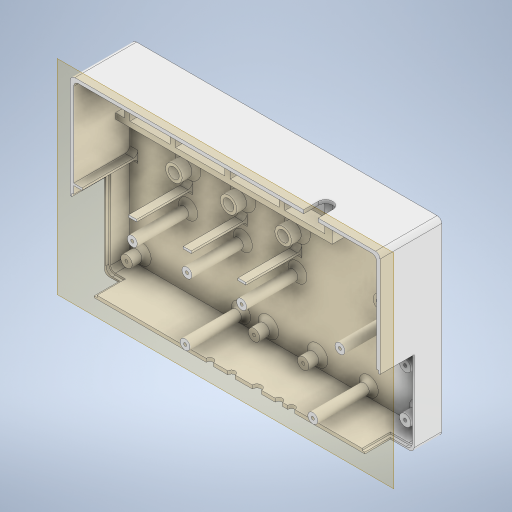
# Autodesk Inventor part: RV_ES_Bottom
Saved by Autodesk Inventor 2023.3 (Build 273359000, 359)
## iProperties
Created: 2023-07-31
Part Number: RV_ES_Bottom
Material: PC/ABS Plastic
Document SubType Name: Modeling
Designer: atrus
Density: 0.357273 g/cm^3
Appearance: Smooth - White
Author: atrus
Autodesk Inventor part; units mm, degrees
ref_plane "YZ Plane" through (0, 0, 0) normal (1, 0, 0) x (0, 1, 0)
ref_plane "XZ Plane" through (0, 0, 0) normal (0, 1, 0) x (-1, 0, 0)
ref_plane "XY Plane" through (0, 0, 0) normal (0, 0, 1) x (1, 0, 0)
sketch "Sketch1" plane through (0, 0, 0) normal (0, 0, 1) x (1, 0, 0)
  line L0 (0, 0) -> (215.9, 0)
  line L1 (215.9, 0) -> (215.9, 132.08)
  line L2 (215.9, 132.08) -> (0, 132.08)
  line L3 (0, 132.08) -> (0, 0)
  dimension "d0" = 215.9
  dimension "d1" = 132.08
  constraints: 8 end point, 2 parallel, 1 horizontal, 1 perpendicular
  measures "d0" distance of L1.end L2.end
  measures "d1" distance of L0.end L1.end
extrude "BasePlate" add sketch "Sketch1" along normal blind 4
sketch "Sketch2" plane through (0, 0, 4) normal (0, 0, 1) x (1, 0, 0)
  circle A0 centre (10.16, 10.16) radius 1.7 construction
  circle A1 centre (99.06, 10.16) radius 1.7 construction
  circle A2 centre (133.35, 10.16) radius 1.7 construction
  circle A3 centre (204.47, 11.43) radius 1.7 construction
  circle A4 centre (156.21, 123.19) radius 1.7 construction
  circle A5 centre (123.19, 123.19) radius 1.7 construction
  circle A6 centre (80.01, 123.19) radius 1.7 construction
  circle A7 centre (46.99, 123.134) radius 1.7 construction
  circle A8 centre (10.16, 10.16) radius 4
  circle A9 centre (99.06, 10.16) radius 4
  circle A10 centre (133.35, 10.16) radius 4
  circle A11 centre (204.47, 11.43) radius 4
  circle A12 centre (156.21, 123.19) radius 4
  circle A13 centre (123.19, 123.19) radius 4
  circle A14 centre (80.01, 123.19) radius 4
  circle A15 centre (46.99, 123.134) radius 4
  circle A16 centre (8.89, 123.19) radius 1.7 construction
  circle A17 centre (8.89, 123.19) radius 4
  circle A18 centre (204.47, 44.45) radius 4
  circle A19 centre (204.47, 44.45) radius 1.7 construction
  point P0 (0, 0)
  dimension "d4" = 8
  constraints: 11 centre point, 9 equal radius, 1 coincident, 2 other
  measures "d4" diameter of A8
ref_plane "Work Plane1" through (212.09, 125.73, 14) normal (0, 0, -1) x (0.0000001, -1, 0)
extrude "PCB Screw Bosses" add sketch "Sketch2" along normal up to surface (10 mm away)
sketch "Sketch3" plane through (0, 0, 4) normal (0, 0, 1) x (1, 0, 0)
  line L0 (0, 0) -> (215.9, 0)
  line L1 (215.9, 0) -> (215.9, 132.08)
  line L2 (215.9, 132.08) -> (0, 132.08)
  line L3 (0, 132.08) -> (0, 0)
  line L4 (213.487, 129.667) -> (213.487, 2.413)
  line L5 (213.487, 2.413) -> (2.413, 2.413)
  line L6 (2.413, 2.413) -> (2.413, 129.667)
  line L7 (2.413, 129.667) -> (213.487, 129.667)
  point P0 (0, 132.08)
  point P1 (215.9, 0)
  dimension "d7" = 2.413
  constraints: 16 end point, 4 parallel, 2 perpendicular, 1 horizontal, 3 other
  measures "d7" distance between parallel lines of L1 L4
extrude "OuterCaseWall" add sketch "Sketch3" along normal blind 15.24
sketch "Sketch4" plane through (0, 0, 4) normal (0, 0, 1) x (1, 0, 0)
  line L0 (2.413, 129.667) -> (2.413, 2.413) projected
  line L1 (153.543, 93.8851) -> (153.543, 92.202)
  line L2 (153.543, 92.202) -> (2.413, 92.202)
  line L3 (2.413, 92.202) -> (2.413, 96.012)
  line L4 (153.543, 115.9189) -> (153.543, 117.602)
  line L5 (153.543, 117.602) -> (2.413, 117.602)
  line L6 (2.413, 117.602) -> (2.413, 113.792)
  line L7 (2.413, 129.667) -> (213.487, 129.667) projected
  line L8 (44.323, 96.012) -> (44.323, 113.792)
  line L9 (40.513, 113.792) -> (40.513, 96.012)
  line L10 (82.423, 96.012) -> (82.423, 113.792)
  line L11 (78.613, 113.792) -> (78.613, 96.012)
  line L12 (120.523, 96.012) -> (120.523, 113.792)
  line L13 (116.713, 113.792) -> (116.713, 96.012)
  line L14 (148.463, 113.792) -> (148.463, 96.012)
  line L15 (153.543, 93.5809) -> (153.543, 115.9189)
  line L16 (8.763, 96.012) -> (8.763, 113.792)
  line L17 (12.573, 113.792) -> (12.573, 96.012)
  line L18 (2.413, 96.012) -> (8.763, 96.012)
  line L19 (12.573, 96.012) -> (40.513, 96.012)
  line L20 (44.323, 96.012) -> (78.613, 96.012)
  line L21 (44.323, 113.792) -> (78.613, 113.792)
  line L22 (2.413, 113.792) -> (8.763, 113.792)
  line L23 (12.573, 113.792) -> (40.513, 113.792)
  line L24 (82.423, 113.792) -> (116.713, 113.792)
  line L25 (120.523, 113.792) -> (148.463, 113.792)
  line L26 (82.423, 96.012) -> (116.713, 96.012)
  line L27 (120.523, 96.012) -> (148.463, 96.012)
  point P0 (0, 0)
  point P1 (2.413, 115.697)
  point P2 (2.413, 94.107)
  point P3 (2.413, 117.602)
  point P4 (2.413, 92.202)
  point P5 (153.543, 93.8851)
  dimension "d10" = 13.97
  dimension "d11" = 21.59
  dimension "d12" = 3.81
  dimension "d13" = 6.35
  dimension "d14" = 151.13
  dimension "d15" = 3.81
  dimension "d16" = 3.81
  dimension "d17" = 3.81
  dimension "d18" = 3.81
  dimension "d19" = 3.81
  dimension "d20" = 27.94
  dimension "d21" = 34.29
  dimension "d22" = 34.29
  dimension "d23" = 27.94
  constraints: 52 end point, 17 parallel, 10 horizontal, 10 perpendicular, 8 collinear, 4 equal length, 2 midpoint, 2 point on line
  measures "d10" distance from line of point (2.413, 115.697) L7
  measures "d11" distance of point (2.413, 115.697) point (2.413, 94.107)
  measures "d12" distance between parallel lines of L17 L16
  measures "d13" distance between parallel lines of L0 L16
  measures "d14" distance of L4.end L5.end
  measures "d15" distance between parallel lines of L9 L8
  measures "d16" distance between parallel lines of L10 L11
  measures "d17" distance between parallel lines of L12 L13
  measures "d18" distance between parallel lines of L5 L23
  measures "d19" distance between parallel lines of L2 L19
  measures "d20" distance between parallel lines of L17 L9
  measures "d21" distance between parallel lines of L8 L11
  measures "d22" distance between parallel lines of L10 L13
  measures "d23" distance between parallel lines of L14 L12
extrude "ReceptBottomRibs" add sketch "Sketch4" along normal up to surface (10 mm away) contours L5 L4 L15 L1 L2 L0 L18 L16 L22
sketch "Sketch5" plane through (0, 0, 4) normal (0, 0, 1) x (1, 0, 0)
  line L0 (54.2784, 65.754) -> (31.8784, 65.754) construction
  line L1 (31.8784, 68.754) -> (54.2784, 68.754) construction
  line L2 (77.7501, 59.2541) -> (77.7501, 75.2541) construction
  line L3 (85.3501, 75.2541) -> (85.3501, 59.2541) construction
  line L4 (70.08, 68.754) -> (92.48, 68.754) construction
  line L5 (92.48, 65.754) -> (70.08, 65.754) construction
  line L6 (3.81, 68.5117) -> (19.05, 68.5117) construction
  line L7 (19.0355, 65.9695) -> (3.81, 65.9695) construction
  line L8 (9.1501, 75.2541) -> (9.1501, 59.2541) construction
  line L9 (39.6501, 59.2541) -> (39.6501, 75.2541) construction
  line L10 (47.2501, 75.2541) -> (47.2501, 59.2541) construction
  line L11 (115.8501, 59.2541) -> (115.8501, 75.2541) construction
  line L12 (123.4501, 75.2541) -> (123.4501, 59.2541) construction
  line L13 (130.58, 65.754) -> (108.18, 65.754) construction
  line L14 (108.18, 68.754) -> (130.58, 68.754) construction
  line L15 (172.95, 68.754) -> (195.35, 68.754) construction
  line L16 (195.35, 65.754) -> (172.95, 65.754) construction
  line L17 (182.51, 53.454) -> (182.51, 105.854) construction
  line L18 (2.413, 92.202) -> (2.413, 2.413) projected
  line L19 (2.413, 68.0117) -> (8.1501, 68.0117)
  line L20 (8.1501, 68.0117) -> (8.1501, 66.4695)
  line L21 (8.1501, 66.4695) -> (2.413, 66.4695)
  line L22 (2.413, 66.4695) -> (2.413, 68.0117)
  line L23 (40.6501, 68.0117) -> (46.2501, 68.0117)
  line L24 (46.2501, 68.0117) -> (46.2501, 66.4695)
  line L25 (46.2501, 66.4695) -> (40.6501, 66.4695)
  line L26 (40.6501, 66.4695) -> (40.6501, 68.0117)
  line L27 (78.7501, 68.0117) -> (84.3501, 68.0117)
  line L28 (84.3501, 68.0117) -> (84.3501, 66.4695)
  line L29 (84.3501, 66.4695) -> (78.7501, 66.4695)
  line L30 (78.7501, 66.4695) -> (78.7501, 68.0117)
  line L31 (116.8501, 68.0117) -> (122.4501, 68.0117)
  line L32 (122.4501, 68.0117) -> (122.4501, 66.4695)
  line L33 (122.4501, 66.4695) -> (116.8501, 66.4695)
  line L34 (116.8501, 66.4695) -> (116.8501, 68.0117)
  line L35 (183.51, 66.4695) -> (194.85, 66.4695)
  line L36 (194.85, 66.4695) -> (194.85, 68.0117)
  line L37 (194.85, 68.0117) -> (183.51, 68.0117)
  line L38 (183.51, 68.0117) -> (183.51, 66.4695)
  point P0 (0, 0)
  dimension "d26" = 0.5
  dimension "d27" = 0.5
  dimension "d28" = 1
  dimension "d29" = 1
  dimension "d30" = 1
  dimension "d31" = 1
  dimension "d32" = 1
  dimension "d33" = 1
  dimension "d34" = 1
  dimension "d35" = 1
  dimension "d36" = 0.5
  constraints: 40 end point, 10 parallel, 9 point on line, 5 horizontal, 5 perpendicular
  measures "d26" distance between parallel lines of L6 L19
  measures "d27" distance between parallel lines of L7 L21
  measures "d28" distance between parallel lines of L8 L20
  measures "d29" distance between parallel lines of L9 L26
  measures "d30" distance from line of L10 L24.end
  measures "d31" distance between parallel lines of L2 L30
  measures "d32" distance between parallel lines of L3 L28
  measures "d33" distance between parallel lines of L11 L34
  measures "d34" distance between parallel lines of L12 L32
  measures "d35" distance between parallel lines of L17 L38
  measures "d36" distance from line of L15.end L36
ref_plane "Top Of Case" through (17.5673, 114.3074, 42.9916) normal (0, 0, 1) x (1, 0, 0)
ref_plane "Offset Top Of Case" through (17.5673, 114.3074, 42.7916) normal (0, 0, 1) x (1, 0, 0)
extrude "Barriers" add sketch "Sketch5" along normal up to surface (38.9916 mm away) contours L19 L20 L21 L18 | L23 L24 L25 L26 | L27 L28 L29 L30 | L31 L32 L33 L34
sketch "Sketch6" plane through (0, 0, 4) normal (0, 0, 1) x (1, 0, 0)
  circle A0 centre (29.21, 123.19) radius 3.75 projected
  circle A1 centre (90.17, 123.19) radius 3.75 projected
  circle A2 centre (113.03, 123.19) radius 3.75 projected
  circle A3 centre (181.61, 123.19) radius 3.75 projected
  circle A4 centre (187.96, 73.66) radius 3.75 projected
  circle A5 centre (119.38, 80.01) radius 3.75 projected
  circle A6 centre (81.28, 80.01) radius 3.75 projected
  circle A7 centre (43.18, 80.01) radius 3.75 projected
  circle A8 centre (29.21, 123.19) radius 5.75
  circle A9 centre (90.17, 123.19) radius 5.75
  circle A10 centre (113.03, 123.19) radius 5.75
  circle A11 centre (181.61, 123.19) radius 5.75
  circle A12 centre (187.96, 73.66) radius 5.75
  circle A13 centre (119.38, 80.01) radius 5.75
  circle A14 centre (81.28, 80.01) radius 5.75
  circle A15 centre (43.18, 80.01) radius 5.75
  dimension "d52" = 2
  constraints: 8 centre point, 7 equal radius
  measures "d52" radial gap between concentric circles of A0 A8
extrude "HVSideBosses" add sketch "Sketch6" along normal up to surface (10 mm away)
sketch "Sketch7" plane through (0, 0, 0) normal (0, 0, -1) x (-1, 0, 0)
  circle A0 centre (-81.28, 80.01) radius 3.75 projected
  circle A1 centre (-29.21, 123.19) radius 3.75 projected
  circle A2 centre (-90.17, 123.19) radius 3.75 projected
  circle A3 centre (-113.03, 123.19) radius 3.75 projected
  circle A4 centre (-181.61, 123.19) radius 3.75 projected
  circle A5 centre (-43.18, 80.01) radius 3.75 construction
  circle A6 centre (-81.28, 80.01) radius 3.75 construction
  circle A7 centre (-119.38, 80.01) radius 3.75 construction
  circle A8 centre (-187.96, 73.66) radius 3.75 construction
  point P0 (0, 0)
  constraints: 5 coincident
hole "HotSideHoles" at (81.28, 80.01, 0) at (29.21, 123.19, 0) at (90.17, 123.19, 0) at (113.03, 123.19, 0) at (181.61, 123.19, 0) at (43.18, 80.01, 0) at (119.38, 80.01, 0) at (187.96, 73.66, 0) direction (0, 0, 1) diameter 3.2766 end through all counterbore diameter 7.62 counterbore depth 3 clearance for "Flat Head Machine Screw (82)" size "#4" standard "Ansi Unified Screw Threads"
chamfer "HotSideHoleChamfer" distance 2.032 angle 45 8 edges at (81.28, 76.2, 3) (90.17, 119.38, 3) (113.03, 119.38, 3) (181.61, 119.38, 3) (29.21, 119.38, 3) (187.96, 69.85, 3) (119.38, 76.2, 3) (43.18, 76.2, 3)
sketch "Sketch8" plane through (0, 0, 4) normal (0, 0, 1) x (1, 0, 0)
  circle A0 centre (169.052, 9.398) radius 3.45
  circle A1 centre (80.01, 9.398) radius 3.45
  circle A2 centre (81.28, 53.34) radius 3.45
  circle A3 centre (119.38, 53.34) radius 3.45
  circle A4 centre (187.96, 60.96) radius 3.45
  circle A5 centre (43.18, 53.34) radius 3.45
  circle A6 centre (169.052, 9.398) radius 3.75 projected
  circle A7 centre (187.96, 60.96) radius 3.75 projected
  circle A8 centre (119.38, 53.34) radius 3.75 projected
  circle A9 centre (81.28, 53.34) radius 3.75 projected
  circle A10 centre (43.18, 53.34) radius 3.75 projected
  circle A11 centre (80.01, 9.398) radius 3.75 projected
  point P0 (0, 0)
  dimension "d53" = 0.3
  constraints: 6 centre point, 6 coincident, 5 equal radius
  measures "d53" radial gap between concentric circles of A10 A5
extrude "LogicSideBosses" add sketch "Sketch8" along normal up to surface (38.9916 mm away) contours A0 | A1 | A2 | A3 | A4 | A5
sketch "Sketch9" plane through (81.28, 53.34, 42.9916) normal (0, 0, 1) x (1, 0, 0)
  circle A0 centre (-38.1, 0) radius 3.45 construction
  circle A1 centre (0, 0) radius 3.45 construction
  circle A2 centre (38.1, 0) radius 3.45 construction
  circle A3 centre (106.68, 7.62) radius 3.45 construction
  circle A4 centre (87.772, -43.942) radius 3.45 construction
  circle A5 centre (17.78, -43.18) radius 4
  circle A6 centre (-1.27, -43.942) radius 3.45 construction
  point P0 (-81.28, -53.34)
  constraints: 1 centre point
hole "LogicSideHoles" at (43.18, 53.34, 42.9916) at (81.28, 53.34, 42.9916) at (119.38, 53.34, 42.9916) at (187.96, 60.96, 42.9916) at (169.052, 9.398, 42.9916) at (80.01, 9.398, 42.9916) direction (0, 0, -1) diameter 2.1565 depth 17.78 tip angle 118 thread size "4-40 UNC" class "2B" standard "ANSI Unified Screw Threads"
fillet "Fillet1" radius 3.175 29 edges at (39.73, 53.34, 4) (77.83, 53.34, 4) (115.93, 53.34, 4) (76.56, 9.398, 4) (165.602, 9.398, 4) (184.51, 60.96, 4) (119.6501, 66.4695, 4) (81.5501, 66.4695, 4) (43.4501, 66.4695, 4) (113.63, 80.01, 4) (119.6501, 68.0117, 4) (75.53, 80.01, 4) (81.5501, 68.0117, 4) (37.43, 80.01, 4) (43.4501, 68.0117, 4) (5.2815, 68.0117, 4) (5.2815, 66.4695, 4) (42.99, 123.134, 4) (76.01, 123.19, 4) (119.19, 123.19, 4) (4.89, 123.19, 4) (175.86, 123.19, 4) (152.21, 123.19, 4) (29.21, 128.94, 4) (6.16, 10.16, 4) (95.06, 10.16, 4) (129.35, 10.16, 4) (200.47, 11.43, 4) (200.47, 44.45, 4)
sketch "Sketch10" plane through (46.99, 123.134, 14) normal (0, 0, 1) x (1, 0, 0)
  circle A0 centre (-38.1, 0.056) radius 4 projected
  circle A1 centre (0, 0) radius 4 projected
  circle A2 centre (33.02, 0.056) radius 4 projected
  circle A3 centre (76.2, 0.056) radius 4 projected
  circle A4 centre (109.22, 0.056) radius 4 projected
  circle A5 centre (157.48, -111.704) radius 4 projected
  circle A6 centre (86.36, -112.974) radius 4 projected
  circle A7 centre (52.07, -112.974) radius 4 projected
  circle A8 centre (-36.83, -112.974) radius 4 projected
  line L0 (-44.577, -120.721) -> (166.497, -120.721) projected
  line L1 (166.497, -120.721) -> (166.497, 6.533) projected
  line L2 (166.497, 6.533) -> (140.7604, 6.533) projected
  line L3 (106.553, -6.6049) -> (106.553, -30.932) projected
  line L4 (106.553, -30.932) -> (-44.577, -30.932) projected
  line L5 (-44.577, -30.932) -> (-44.577, -51.9474) projected
  line L6 (-38.8399, -51.9474) -> (-38.8399, -59.8395) projected
  line L7 (-44.577, -59.8395) -> (-44.577, -120.721) projected
  line L8 (37.3601, -51.9474) -> (37.3601, -59.8395) projected
  line L9 (31.7601, -59.8395) -> (31.7601, -51.9474) projected
  circle A9 centre (140.97, -49.474) radius 5.75 projected
  line L10 (75.4601, -51.9474) -> (75.4601, -59.8395) projected
  line L11 (69.8601, -59.8395) -> (69.8601, -51.9474) projected
  line L12 (-0.7399, -51.9474) -> (-0.7399, -59.8395) projected
  line L13 (-6.3399, -59.8395) -> (-6.3399, -51.9474) projected
  circle A10 centre (157.48, -78.684) radius 1.7 projected
  line L14 (-44.577, 6.533) -> (-44.577, 3.1429) projected
  line L15 (-33.5995, -5.532) -> (-24.7392, -5.532) projected
  line L16 (-10.8208, -5.532) -> (-4.5692, -5.532) projected
  line L17 (4.5692, -5.532) -> (28.5195, -5.532) projected
  arc A11 (44.5353, -5.532) -> (39.0064, 4.0112) centre (43.18, 0.056) ccw projected
  line L18 (44.5353, -5.532) -> (64.6847, -5.532) projected
  arc A12 (70.2136, 4.0112) -> (64.6847, -5.532) centre (66.04, 0.056) ccw projected
  line L19 (-38.227, -9.342) -> (-44.577, -9.342) projected
  line L20 (-44.577, -27.122) -> (-38.227, -27.122) projected
  line L21 (-38.227, -27.122) -> (-38.227, -9.342) projected
  line L22 (-44.577, -3.0309) -> (-44.577, -5.532) projected
  line L23 (-44.577, -9.342) -> (-44.577, -27.122) projected
  arc A13 (29.9331, 6.533) -> (28.5195, -5.532) centre (33.02, 0.056) ccw projected
  line L24 (29.9331, 6.533) -> (2.9666, 6.533) projected
  arc A14 (4.5692, -5.532) -> (2.9666, 6.533) centre (0, 0) ccw projected
  arc A15 (73.1131, 6.533) -> (70.2136, 4.0112) centre (76.2, 0.056) ccw projected
  line L25 (73.1131, 6.533) -> (36.1069, 6.533) projected
  arc A16 (39.0064, 4.0112) -> (36.1069, 6.533) centre (33.02, 0.056) ccw projected
  arc A17 (-41.1869, 6.533) -> (-44.577, 3.1429) centre (-38.1, 0.056) ccw projected
  line L26 (-41.1869, 6.533) -> (-44.577, 6.533) projected
  arc A18 (-44.577, -3.0309) -> (-42.6005, -5.532) centre (-38.1, 0.056) ccw projected
  line L27 (-44.577, -5.532) -> (-42.6005, -5.532) projected
  arc A19 (-10.8208, -5.532) -> (-11.6396, 6.533) centre (-17.78, 0.056) ccw projected
  arc A20 (-2.9666, 6.533) -> (-4.5692, -5.532) centre (0, 0) ccw projected
  line L28 (-2.9666, 6.533) -> (-11.6396, 6.533) projected
  arc A21 (-23.9204, 6.533) -> (-24.7392, -5.532) centre (-17.78, 0.056) ccw projected
  line L29 (-23.9204, 6.533) -> (-35.0131, 6.533) projected
  arc A22 (-33.5995, -5.532) -> (-35.0131, 6.533) centre (-38.1, 0.056) ccw projected
  circle A23 centre (-36.83, -112.974) radius 7.175 projected
  arc A24 (128.4796, 6.533) -> (140.7604, 6.533) centre (134.62, 0.056) ccw projected
  line L30 (128.4796, 6.533) -> (112.3069, 6.533) projected
  arc A25 (106.553, -6.6049) -> (112.3069, 6.533) centre (109.22, 0.056) ccw projected
  line L31 (-38.8399, -51.9474) -> (-44.577, -51.9474) projected
  line L32 (-44.577, -59.8395) -> (-38.8399, -59.8395) projected
  line L33 (31.7601, -59.8395) -> (37.3601, -59.8395) projected
  line L34 (32.9468, -51.9474) -> (31.7601, -51.9474) projected
  arc A26 (35.6332, -51.9474) -> (32.9468, -51.9474) centre (34.29, -43.124) ccw projected
  line L35 (37.3601, -51.9474) -> (35.6332, -51.9474) projected
  circle A27 centre (140.97, -62.174) radius 6.625 projected
  line L36 (69.8601, -59.8395) -> (75.4601, -59.8395) projected
  line L37 (71.0467, -51.9474) -> (69.8601, -51.9474) projected
  arc A28 (73.7333, -51.9474) -> (71.0467, -51.9474) centre (72.39, -43.124) ccw projected
  line L38 (75.4601, -51.9474) -> (73.7333, -51.9474) projected
  line L39 (-6.3399, -59.8395) -> (-0.7399, -59.8395) projected
  line L40 (-5.1533, -51.9474) -> (-6.3399, -51.9474) projected
  arc A29 (-2.4667, -51.9474) -> (-5.1533, -51.9474) centre (-3.81, -43.124) ccw projected
  line L41 (-0.7399, -51.9474) -> (-2.4667, -51.9474) projected
  point P0 (-46.99, -123.134)
hole "PCBMountHoles" at (46.99, 123.134, 14) at (8.89, 123.19, 14) at (80.01, 123.19, 14) at (123.19, 123.19, 14) at (156.21, 123.19, 14) at (10.16, 10.16, 14) at (99.06, 10.16, 14) at (133.35, 10.16, 14) at (204.47, 11.43, 14) at (204.47, 44.45, 14) direction (0, 0, -1) diameter 2.1565 end through all thread size "4-40 UNC" class "2B" standard "ANSI Unified Screw Threads"
sketch "Sketch11" plane through (0, 0, 19.24) normal (0, 0, 1) x (1, 0, 0)
  line L0 (2.413, 59.2541) -> (2.413, 129.667) projected
  line L1 (2.413, 59.2541) -> (2.413, 129.667)
  line L2 (2.413, 129.667) -> (213.487, 129.667) projected
  line L3 (2.413, 129.667) -> (213.487, 129.667)
  line L4 (213.487, 129.667) -> (213.487, 59.2541)
  line L5 (213.487, 129.667) -> (213.487, 2.413) projected
  line L6 (215.9, 0) -> (215.9, 132.08) projected
  line L7 (215.9, 59.2541) -> (215.9, 132.08)
  line L8 (215.9, 132.08) -> (0, 132.08)
  line L9 (0, 132.08) -> (0, 59.2541)
  line L10 (0, 132.08) -> (0, 0) projected
  line L11 (2.413, 59.2541) -> (0, 59.2541)
  line L12 (213.487, 59.2541) -> (215.9, 59.2541)
  line L13 (9.1501, 59.2541) -> (39.6501, 59.2541) construction
  point P0 (2.413, 66.4695)
  point P1 (1.2065, 59.2541)
  constraints: 16 end point, 3 point on line, 2 collinear, 2 horizontal, 2 horizontal alignment, 2 vertical, 1 midpoint, 1 perpendicular
extrude "HV Upper Wall" add sketch "Sketch11" along normal up to surface (23.7516 mm away)
sketch "Sketch12" plane through (0, 132.08, 0) normal (0, 1, 0) x (1, 0, 0)
  line L0 (213.487, -42.9916) -> (2.413, -42.9916) projected
  line L1 (172.72, -42.9916) -> (172.72, -32.7516)
  line L2 (167.72, -27.7516) -> (167.72, -27.7516)
  line L3 (162.72, -32.7516) -> (162.72, -42.9916)
  line L4 (215.9, 0) -> (215.9, -42.9916) projected
  arc A0 (167.72, -27.7516) -> (162.72, -32.7516) centre (167.72, -32.7516) ccw
  arc A1 (172.72, -32.7516) -> (167.72, -27.7516) centre (167.72, -32.7516) ccw
  point P0 (0, 0)
  point P1 (172.72, -27.7516)
  point P2 (162.72, -27.7516)
  point P3 (172.72, -37.8716)
  dimension "d74" = 10
  dimension "d75" = 43.18
  dimension "d76" = 15.24
  dimension "d77" = 5
  constraints: 6 end point, 6 point on line, 4 point on circle, 4 tangent, 2 centre point, 2 perpendicular, 1 concentric, 1 midpoint, 1 vertical
  measures "d74" distance of point (172.72, -27.752) point (162.72, -27.752)
  measures "d75" distance from line of L4 point (172.72, -37.872)
  measures "d76" distance of point (162.72, -27.752) L3.end
  measures "d77" radius of A0
extrude "Cord cut" cut sketch "Sketch12" against normal blind 25.4
fillet "HV Corner Fillets" radius 3.175 4 edges at (0, 132.08, 21.4958) (213.487, 129.667, 23.4958) (215.9, 132.08, 21.4958) (2.413, 129.667, 23.4958)
sketch "Sketch13" plane through (187.96, 73.66, 14) normal (0, 0, 1) x (1, 0, 0)
  line L0 (-65.5099, -5.6483) -> (-65.5099, -7.1905) construction
  line L1 (25.527, -71.247) -> (25.527, 52.832) construction
  line L2 (-4.3589, -6.075) -> (-4.3589, -3.75)
  line L3 (-4.3589, -3.75) -> (4.3589, -3.75)
  line L4 (4.3589, -3.75) -> (4.3589, -6.075)
  line L5 (4.3589, -6.075) -> (-4.3589, -6.075)
  circle A0 centre (0, 0) radius 5.75 projected
  circle A1 centre (0, 0) radius 3.75 projected
  circle A2 centre (0, -12.7) radius 6.625 construction
  point P0 (-187.96, -73.66)
  point P1 (0, -3.75)
  constraints: 8 end point, 2 point on circle, 2 vertical, 1 midpoint, 1 parallel, 1 perpendicular, 1 tangent, 1 vertical alignment, 1 other
extrude "BossCutPowerSupply" cut sketch "Sketch13" against normal up to surface (10 mm away) contours L2 A0 L4 L5 | L3 A0 picked at (2.5581, -4.066)
fillet "LgicCornerFillets" radius 3.175 4 edges at (0, 0, 9.62) (215.9, 0, 9.62) (2.413, 2.413, 11.62) (213.487, 2.413, 11.62)
sketch "Sketch14" plane through (0, 0, 19.24) normal (0, 0, 1) x (1, 0, 0)
  circle A0 centre (80.01, 9.398) radius 1.0782 construction
  circle A1 centre (80.01, 9.398) radius 3.45 construction
  line L0 (151.92, 16.9397) -> (151.92, 21.3401) construction
  line L1 (84.975, 21.3101) -> (84.975, 16.9097) construction
  line L2 (5.588, 2.413) -> (210.312, 2.413) projected
  line L3 (3.175, 0) -> (212.725, 0) projected
  line L4 (10.668, 2.413) -> (199.39, 2.413)
  line L5 (199.39, 2.413) -> (199.39, 0)
  line L6 (199.39, 0) -> (10.668, 0)
  line L7 (10.668, 0) -> (10.668, 2.413)
  circle A2 centre (204.47, 11.43) radius 1.0782 construction
  point P0 (0, 0)
  point P1 (199.39, 1.2065)
  point P2 (151.92, 19.1399)
  point P3 (10.668, 1.2065)
  point P4 (84.975, 19.1099)
  point P5 (10.668, 0)
  point P6 (199.39, 2.413)
  dimension "d95" = 5.08
  dimension "d96" = 5.08
  constraints: 8 end point, 4 midpoint, 2 parallel, 2 point on line, 1 horizontal, 1 perpendicular
  measures "d95" horizontal distance of point (199.39, 1.206) A2.centre
  measures "d96" horizontal distance of L2.start point (10.668, 1.206)
extrude "Extrusion11" add sketch "Sketch14" along normal blind 17.78
sketch "Sketch15" plane through (3.175, 0, 0) normal (0, -1, 0) x (1, 0, 0)
  line L0 (7.493, 37.02) -> (196.215, 37.02) projected
  circle A0 centre (88.11, 37.02) radius 2.54
  circle A1 centre (103.2, 37.02) radius 2.54
  circle A2 centre (120.915, 37.02) radius 3.175
  circle A3 centre (136.155, 37.02) radius 2.54
  circle A4 centre (144.945, 37.02) radius 2.54
  line L1 (88.26, 22.2733) -> (89.674, 22.2733) construction
  ellipse E0 centre (88.86, 23.1218) end of major axis (90.31, 23.1218) minor radius 1.0253 (89.674, 22.2733) -> (89.76, 22.3179) ccw construction
  line L2 (89.76, 22.3179) -> (89.76, 23.9257) construction
  ellipse E1 centre (88.86, 23.1218) end of major axis (90.31, 23.1218) minor radius 1.0253 (89.76, 23.9257) -> (89.674, 23.9704) ccw construction
  line L3 (89.674, 23.9704) -> (88.86, 23.9704) construction
  line L4 (88.86, 23.9704) -> (88.26, 23.9704) construction
  line L5 (88.26, 23.9704) -> (88.26, 22.2733) construction
  line L6 (103.5, 22.2733) -> (104.914, 22.2733) construction
  ellipse E2 centre (104.1, 23.1218) end of major axis (105.55, 23.1218) minor radius 1.0253 (104.914, 22.2733) -> (105, 22.3179) ccw construction
  line L7 (105, 22.3179) -> (105, 23.9257) construction
  ellipse E3 centre (104.1, 23.1218) end of major axis (105.55, 23.1218) minor radius 1.0253 (105, 23.9257) -> (104.914, 23.9704) ccw construction
  line L8 (104.914, 23.9704) -> (104.1, 23.9704) construction
  line L9 (104.1, 23.9704) -> (103.5, 23.9704) construction
  line L10 (103.5, 23.9704) -> (103.5, 22.2733) construction
  line L11 (140.115, 28.8269) -> (137.325, 28.8269) construction
  point P0 (-3.175, 0)
  point P1 (144.945, 28.8269)
  point P2 (88.11, 26.7147)
  point P3 (103.2, 27.1269)
  point P4 (120.915, 27.1269)
  point P5 (136.155, 26.6735)
  point P6 (147.485, 37.02)
  point P7 (142.405, 37.02)
  point P8 (124.09, 37.02)
  point P9 (117.74, 37.02)
  point P10 (105.74, 37.02)
  point P11 (100.66, 37.02)
  point P12 (90.65, 37.02)
  point P13 (85.57, 37.02)
  dimension "d90" = 5.08
  dimension "d91" = 6.35
  dimension "d92" = 5.08
  constraints: 5 centre point, 5 point on line, 5 vertical alignment, 2 equal radius, 10 other
  measures "d90" diameter of A0
  measures "d91" diameter of A2
  measures "d92" diameter of A3
extrude "Extrusion12" cut sketch "Sketch15" against normal blind 19.05 contours L0 A0 | L0 A1 | L0 A2 | A3 L0 | L0 A3 | L0 A4 picked at (88.2121, 36.1795) picked at (103.3021, 36.1795) picked at (120.0921, 36.0649) picked at (144.3481, 35.3683)
sketch "Sketch16" plane through (0, 0, 19.24) normal (0, 0, 1) x (1, 0, 0)
  line L0 (10.668, 2.413) -> (5.588, 2.413) projected
  arc A0 (2.413, 5.588) -> (5.588, 2.413) centre (5.588, 5.588) ccw projected
  line L1 (2.413, 5.588) -> (2.413, 59.2541) projected
  line L2 (1.113, 59.2541) -> (1.113, 5.588)
  arc A1 (1.113, 5.588) -> (5.588, 1.113) centre (5.588, 5.588) ccw
  line L3 (5.588, 1.113) -> (10.668, 1.113)
  line L4 (2.413, 59.2541) -> (0, 59.2541) projected
  line L5 (1.113, 59.2541) -> (2.413, 59.2541)
  line L6 (10.668, 0) -> (10.668, 2.413) projected
  line L7 (10.668, 2.413) -> (10.668, 1.113)
  line L8 (213.487, 59.2541) -> (213.487, 5.588) projected
  arc A2 (210.312, 2.413) -> (213.487, 5.588) centre (210.312, 5.588) ccw projected
  line L9 (210.312, 2.413) -> (199.39, 2.413) projected
  line L10 (214.787, 59.2541) -> (214.787, 5.588)
  arc A3 (210.312, 1.113) -> (214.787, 5.588) centre (210.312, 5.588) ccw
  line L11 (210.312, 1.113) -> (199.39, 1.113)
  line L12 (215.9, 59.2541) -> (213.487, 59.2541) projected
  line L13 (214.787, 59.2541) -> (213.487, 59.2541)
  line L14 (199.39, 1.113) -> (199.39, 2.413)
  line L15 (5.588, 2.413) -> (210.312, 2.413) projected
  point P0 (0, 0)
  dimension "d97" = 1.3
  dimension "d100" = 1.3
  constraints: 16 end point, 4 point on circle, 2 centre point, 2 perpendicular, 1 collinear, 1 horizontal, 4 other
  measures "d97" distance between parallel lines of L1 L2
  measures "d100" distance between parallel lines of L8 L10
extrude "OuterWallLip" cut sketch "Sketch16" against normal blind 2
sketch "Sketch17" plane through (0, 59.2541, 42.9916) normal (0, -1, 0) x (1, 0, 0)
  line L0 (214.787, -23.7516) -> (214.787, -25.7516) projected
  line L1 (214.787, -23.7516) -> (214.7559, 0)
  line L2 (215.9, 0) -> (213.487, 0) projected
  line L3 (214.7559, 0) -> (213.487, 0)
  line L4 (213.487, 0) -> (213.487, -25.7516)
  line L5 (213.487, -25.7516) -> (214.787, -25.7516)
  line L6 (214.787, -23.7516) -> (214.787, -25.7516)
  line L7 (1.113, -25.7516) -> (2.413, -25.7516) projected
  line L8 (1.113, -25.7516) -> (2.413, -25.7516)
  line L9 (2.413, 0) -> (2.413, -25.7516) projected
  line L10 (2.413, -25.7516) -> (2.413, 0)
  line L11 (1.113, -23.7516) -> (1.113, -25.7516) projected
  line L12 (1.113, -25.7516) -> (1.113, -23.7516)
  line L13 (1.113, -23.7516) -> (1.113, 0)
  line L14 (2.413, 0) -> (0, 0) projected
  line L15 (2.413, 0) -> (1.113, 0)
  point P0 (0, -42.9916)
  constraints: 20 end point, 4 perpendicular, 3 point on line, 1 collinear, 1 horizontal, 1 vertical
extrude "Extrusion14" cut sketch "Sketch17" against normal blind 2
sketch "Sketch18" plane through (199.39, 0, 37.02) normal (1, 0, 0) x (0, 0, -1)
  line L0 (17.78, 1.113) -> (19.78, 1.113) projected
  line L1 (19.78, 1.113) -> (19.78, 2.413) projected
  line L2 (17.78, 1.113) -> (17.78, 0) projected
  line L3 (0, 2.413) -> (19.78, 2.413) projected
  line L4 (19.78, 2.413) -> (0, 2.413)
  line L5 (17.78, 1.113) -> (0, 1.113)
  line L6 (0, 0) -> (0, 2.413) projected
  line L7 (0, 2.413) -> (0, 1.113)
  point P0 (37.02, 0)
  constraints: 6 end point, 1 horizontal, 1 perpendicular, 1 point on line
extrude "Extrusion15" cut sketch "Sketch18" against normal blind 2
sketch "Sketch19" plane through (10.668, 0, 37.02) normal (-1, 0, 0) x (0, 0, 1)
  line L0 (-17.78, 1.113) -> (-19.78, 1.113) projected
  line L1 (-19.78, 2.413) -> (-19.78, 1.113) projected
  line L2 (-19.78, 2.413) -> (0, 2.413) projected
  line L3 (-17.78, 1.113) -> (0, 1.113)
  line L4 (0, 2.413) -> (0, 0) projected
  line L5 (0, 2.413) -> (0, 1.113)
  point P0 (-37.02, 0)
  constraints: 4 end point, 1 horizontal, 1 perpendicular, 1 point on line
extrude "Extrusion16" cut sketch "Sketch19" against normal blind 2
body "Solid1"
